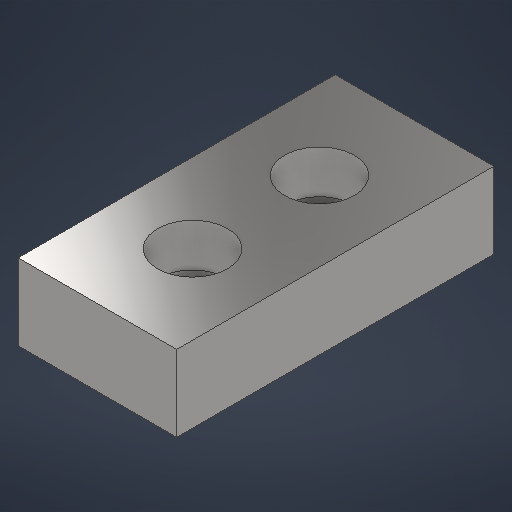
# Autodesk Inventor part: Part5
Saved by Autodesk Inventor 2026 (Build 300175000, 175)
## iProperties
Created: 2026-03-22
Part Number: Part5
Material: Generic
Document SubType Name: Modeling
Designer: Mlinč
Density: 1 g/cm^3
Appearance: Default
Author: Mlinč
Autodesk Inventor part; units mm, degrees
ref_plane "YZ Plane" through (0, 0, 0) normal (1, 0, 0) x (0, 1, 0)
ref_plane "XZ Plane" through (0, 0, 0) normal (0, 1, 0) x (-1, 0, 0)
ref_plane "XY Plane" through (0, 0, 0) normal (0, 0, 1) x (1, 0, 0)
sketch "Sketch1" plane through (0, 0, 0) normal (0, 1, 0) x (-1, 0, 0)
  line L0 (0, 0) -> (25, 0)
  line L1 (25, 0) -> (25, -50)
  line L2 (25, -50) -> (0, -50)
  line L3 (0, -50) -> (0, 0)
  dimension "d0" = 25
  dimension "d1" = 50
  constraints: 8 end point, 2 parallel, 1 horizontal, 1 perpendicular
  measures "d0" distance of L0.start L0.end
  measures "d1" distance of L0.end L1.end
extrude "Extrusion1" add sketch "Sketch1" along normal blind 12
sketch "Sketch2" plane through (0, 12, 0) normal (0, 1, 0) x (1, 0, 0)
  circle A0 centre (-12.5, 15) radius 3.3
  circle A1 centre (-12.5, 35) radius 3.3
  line L0 (-25, 0) -> (0, 0) projected
  line L1 (0, 0) -> (0, 50) projected
  dimension "d4" = 6.6
  dimension "d5" = 20
  dimension "d6" = 15
  dimension "d7" = 12.5
  constraints: 2 centre point, 1 equal radius, 1 vertical alignment
  measures "d4" diameter of A0
  measures "d5" distance of A1.centre A0.centre
  measures "d6" distance from line of L0 A0.centre
  measures "d7" distance from line of L1 A0.centre
extrude "Extrusion2" cut sketch "Sketch2" against normal through all
sketch "Sketch3" plane through (0, 12, 0) normal (0, 1, 0) x (1, 0, 0)
  circle A0 centre (-12.5, 15) radius 3.3 projected
  circle A1 centre (-12.5, 15) radius 5.5
  circle A2 centre (-12.5, 35) radius 3.3 projected
  circle A3 centre (-12.5, 35) radius 5.5
  point P0 (0, 0)
  dimension "d10" = 11
  constraints: 2 centre point, 2 coincident, 1 equal radius
  measures "d10" diameter of A1
extrude "Extrusion3" cut sketch "Sketch3" against normal blind 6.8 contours A0 | A1 | A2 | A3
body "Solid1"
